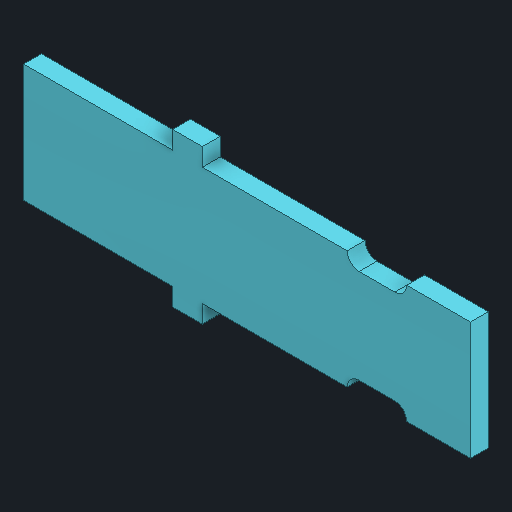
# Autodesk Inventor part: tibea_reinforcment2_steel
Saved by Autodesk Inventor 2026 (Build 300175000, 175)
## iProperties
Created: 2026-05-02
Part Number: tibea_reinforcment2_steel
Material: Сталь
Document SubType Name: Modeling
Designer: user
Density: 7.85 g/cm^3
Appearance: Серо-синий
Mass: 34.8171 g
Surface Area: 35.7537 cm^2
Volume: 4.4353 cm^3
Author: user
Autodesk Inventor part; units mm, degrees
ref_plane "YZ Plane" through (0, 0, 0) normal (1, 0, 0) x (0, 1, 0)
ref_plane "XZ Plane" through (0, 0, 0) normal (0, 1, 0) x (-1, 0, 0)
ref_plane "XY Plane" through (0, 0, 0) normal (0, 0, 1) x (1, 0, 0)
sketch "Эскиз3" plane through (0, 0, 0) normal (0, 0, 1) x (1, 0, 0)
  line L0 (0, 0) -> (25, 0)
  line L1 (25, 19.8) -> (0, 19.8)
  line L2 (0, 19.8) -> (0, 0)
  line L3 (25, 0) -> (25, -3)
  line L4 (25, -3) -> (30, -3)
  line L5 (30, -3) -> (30, 0)
  line L6 (75, 0) -> (75, 19.8)
  line L7 (30, 19.8) -> (30, 22.8)
  line L8 (30, 22.8) -> (25, 22.8)
  line L9 (25, 22.8) -> (25, 19.8)
  line L10 (62.2966, 2) -> (56.2966, 2)
  line L11 (62.2966, 17.8) -> (56.2966, 17.8)
  arc A0 (54.2966, 19.8) -> (56.2966, 17.8) centre (56.2966, 19.8) ccw
  arc A1 (62.2966, 17.8) -> (64.2966, 19.8) centre (62.2966, 19.8) ccw
  arc A2 (64.2966, 0) -> (62.2966, 2) centre (62.2966, 0) ccw
  arc A3 (56.2966, 2) -> (54.2966, 0) centre (56.2966, 0) ccw
  line L12 (30, 0) -> (54.2966, 0)
  line L13 (64.2966, 0) -> (75, 0)
  line L14 (75, 19.8) -> (64.2966, 19.8)
  line L15 (54.2966, 19.8) -> (30, 19.8)
  line L16 (54.2966, 19.8) -> (54.2966, 19.8)
  line L17 (64.2966, 19.8) -> (64.2966, 19.8)
  point P0 (64.5264, 2)
  point P1 (63.7076, 0)
  point P2 (54.5264, 2)
  point P3 (64.2966, 17.8)
  point P4 (54.2966, 17.8)
  point P5 (63.7076, 1.4173)
  point P6 (54.2966, 19.8)
  point P7 (64.2966, 19.8)
  dimension "d8" = 19.8
  dimension "d9" = 25
  dimension "d10" = 5
  dimension "d11" = 45
  dimension "d12" = 3
  dimension "d13" = 10
  dimension "d15" = 10
  dimension "d16" = 2
  dimension "d17" = 2
  constraints: 36 end point, 11 point on circle, 10 perpendicular, 7 point on line, 7 vertical alignment, 6 horizontal, 5 horizontal alignment, 4 centre point, 4 tangent, 3 equal radius, 3 parallel, 2 coincident, 1 collinear, 1 vertical, 10 other
  measures "d8" distance between parallel lines of L0 L1
  measures "d9" distance between parallel lines of L2 L3
  measures "d10" distance between parallel lines of L3 L5
  measures "d11" distance between parallel lines of L5 L6
  measures "d12" distance of L0.end L3.end
  measures "d13" distance of point (54.526, 2) point (64.526, 2)
  measures "d15" distance of point (64.297, 17.8) point (54.297, 17.8)
  measures "d16" distance of L14.end point (64.297, 17.8)
  measures "d17" radius of A0
extrude "Выдавливание3" add sketch "Эскиз3" along normal blind 3
equation "\"d8\" = width_profile_tibea - 2 * tolerance_plazma"
equation "\"d12\" = thickness_steel"
equation "\"d6\" = thickness_steel"
equation "\"tolerance_plazma\" = 0.1"
equation "\"thickness_steel\" = 3"
equation "\"d_main_screw_holes\" = 6.1"
equation "\"d_main_shaft\" = 15"
equation "\"thickness_profile_tibea\" = 3"
equation "\"hight_shaft_shift\" = 37"
equation "\"thickness_profile_femur\" = 3"
equation "\"width_shaft_shift\" = 35"
equation "\"width_flattened_surface\" = 12"
equation "\"width_profile_tibea\" = 20"
